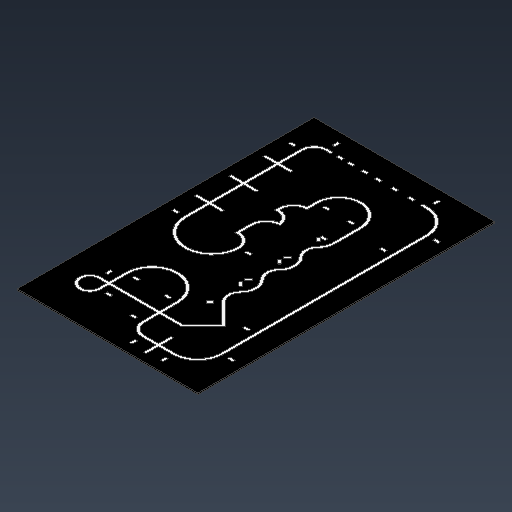
# Autodesk Inventor part: Pista_Teste_V1
Saved by Autodesk Inventor 2026.1 (Build 301233020, 233B)
## iProperties
Created: 2026-04-30
Part Number: Pista_Teste_V1
Material: Genérico
Document SubType Name: Modeling
Designer: celio
Density: 1 g/cm^3
Appearance: Padrão
Author: celio
Autodesk Inventor part; units mm, degrees
ref_plane "YZ Plane" through (0, 0, 0) normal (1, 0, 0) x (0, 1, 0)
ref_plane "XZ Plane" through (0, 0, 0) normal (0, 1, 0) x (-1, 0, 0)
ref_plane "XY Plane" through (0, 0, 0) normal (0, 0, 1) x (1, 0, 0)
sketch "Esboço1" plane through (0, 0, 0) normal (0, 1, 0) x (-1, 0, 0)
  line L0 (0, 0) -> (1320, 0)
  line L1 (1320, 0) -> (1320, -2170)
  line L2 (1320, -2170) -> (0, -2170)
  line L3 (0, -2170) -> (0, 0)
  line L4 (1170, -2020) -> (1170, -150) construction
  line L5 (1170, -150) -> (150, -150) construction
  line L6 (150, -150) -> (150, -2020) construction
  line L7 (150, -2020) -> (1170, -2020) construction
  line L8 (150, -335) -> (150, -1835)
  arc A0 (335, -150) -> (150, -335) centre (335, -335) ccw
  line L9 (150, -335) -> (335, -335) construction
  line L10 (335, -150) -> (335, -335) construction
  arc A1 (660, -250) -> (560, -150) centre (560, -250) ccw
  line L11 (560, -150) -> (560, -250) construction
  line L12 (660, -250) -> (560, -250) construction
  arc A2 (660, -500) -> (1010, -500) centre (835, -500) ccw
  line L13 (660, -500) -> (835, -500) construction
  line L14 (1010, -500) -> (835, -500) construction
  arc A3 (1090, -380) -> (1010, -300) centre (1090, -300) ccw
  line L15 (1010, -300) -> (1090, -300) construction
  line L16 (1090, -380) -> (1090, -300) construction
  line L17 (490, -380) -> (348.5786, -521.4214)
  line L18 (348.5786, -521.4214) -> (490, -662.8427)
  arc A4 (490, -804.2641) -> (490, -662.8427) centre (419.2893, -733.5534) ccw
  line L19 (490, -662.8427) -> (419.2893, -733.5534) construction
  line L20 (490, -804.2641) -> (419.2893, -733.5534) construction
  arc A5 (490, -804.2641) -> (490, -945.6854) centre (560.7107, -874.9747) ccw
  line L21 (490, -804.2641) -> (560.7107, -874.9747) construction
  line L22 (490, -945.6854) -> (560.7107, -874.9747) construction
  arc A6 (490, -1087.1068) -> (490, -945.6854) centre (419.2893, -1016.3961) ccw
  line L23 (490, -945.6854) -> (419.2893, -1016.3961) construction
  line L24 (490, -1087.1068) -> (419.2893, -1016.3961) construction
  arc A7 (490, -1087.1068) -> (490, -1228.5281) centre (560.7107, -1157.8175) ccw
  line L25 (490, -1087.1068) -> (560.7107, -1157.8175) construction
  line L26 (490, -1228.5281) -> (560.7107, -1157.8175) construction
  arc A8 (490, -1369.9495) -> (490, -1228.5281) centre (419.2893, -1299.2388) ccw
  line L27 (490, -1228.5281) -> (419.2893, -1299.2388) construction
  line L28 (490, -1369.9495) -> (419.2893, -1299.2388) construction
  arc A9 (490, -1369.9495) -> (460.7107, -1440.6602) centre (560.7107, -1440.6602) ccw
  line L29 (490, -1369.9495) -> (560.7107, -1440.6602) construction
  line L30 (460.7107, -1440.6602) -> (560.7107, -1440.6602) construction
  line L31 (460.7107, -1440.6602) -> (460.7107, -1640.6602)
  arc A10 (460.7107, -1640.6602) -> (760.7096, -1640.0838) centre (610.7107, -1640.6602) ccw
  arc A11 (1170.7096, -1070.0838) -> (760.7096, -1070.0838) centre (965.7096, -1070.0838) ccw
  line L32 (760.7096, -1070.0838) -> (965.7096, -1070.0838) construction
  line L33 (1170.7096, -1070.0838) -> (965.7096, -1070.0838) construction
  arc A12 (1069.9166, -2020) -> (1170, -1920.0835) centre (1070, -1920) ccw
  line L34 (1170, -1920.0835) -> (1070, -1920) construction
  line L35 (1069.9166, -2020) -> (1070, -1920) construction
  arc A13 (150, -1835) -> (335, -2020) centre (335, -1835) ccw
  line L36 (150, -1835) -> (335, -1835) construction
  line L37 (335, -2020) -> (335, -1835) construction
  line L38 (760.7096, -1640.0838) -> (760.7096, -1560.0838)
  arc A14 (760.7096, -1560.0838) -> (860.7096, -1460.0838) centre (760.7096, -1460.0838) ccw
  arc A15 (760.7096, -1360.0838) -> (860.7096, -1460.0838) centre (860.7096, -1360.0838) ccw
  arc A16 (760.7096, -1360.0838) -> (860.7096, -1260.0838) centre (760.7096, -1260.0838) ccw
  arc A17 (760.7096, -1070.0838) -> (860.7096, -1170.0838) centre (860.7096, -1070.0838) ccw
  line L39 (860.7096, -1170.0838) -> (860.7096, -1260.0838)
  line L40 (1069.9166, -2020) -> (1029.9166, -2020)
  line L41 (1029.9166, -2020) -> (989.9166, -2020) construction
  line L42 (989.9166, -2020) -> (949.9166, -2020)
  line L43 (949.9166, -2020) -> (909.9166, -2020) construction
  line L44 (909.9166, -2020) -> (869.9166, -2020)
  line L45 (869.9166, -2020) -> (809.9166, -2020) construction
  line L46 (809.9166, -2020) -> (769.9166, -2020)
  line L47 (769.9166, -2020) -> (709.9166, -2020) construction
  line L48 (709.9166, -2020) -> (669.9166, -2020)
  line L49 (669.9166, -2020) -> (589.9166, -2020) construction
  line L50 (589.9166, -2020) -> (549.9166, -2020)
  line L51 (549.9166, -2020) -> (469.9166, -2020) construction
  line L52 (469.9166, -2020) -> (429.9166, -2020)
  line L53 (335, -2020) -> (375, -2020)
  line L54 (375, -2000) -> (335, -2000)
  arc A18 (170, -1835) -> (335, -2000) centre (335, -1835) ccw
  line L55 (170, -1835) -> (170, -335)
  arc A19 (335, -170) -> (170, -335) centre (335, -335) ccw
  arc A20 (640, -250) -> (560, -170) centre (560, -250) ccw
  arc A21 (640, -500) -> (1030, -500) centre (835, -500) ccw
  arc A22 (1090, -360) -> (1030, -300) centre (1090, -300) ccw
  line L56 (481.7157, -360) -> (320.2944, -521.4214)
  line L57 (320.2944, -521.4214) -> (475.8579, -676.9848)
  arc A23 (475.8579, -790.1219) -> (475.8579, -676.9848) centre (419.2893, -733.5534) ccw
  arc A24 (475.8579, -790.1219) -> (475.8579, -959.8276) centre (560.7107, -874.9747) ccw
  arc A25 (475.8579, -1072.9646) -> (475.8579, -959.8276) centre (419.2893, -1016.3961) ccw
  arc A26 (475.8579, -1072.9646) -> (475.8579, -1242.6703) centre (560.7107, -1157.8175) ccw
  arc A27 (475.8579, -1355.8074) -> (475.8579, -1242.6703) centre (419.2893, -1299.2388) ccw
  arc A28 (475.8579, -1355.8074) -> (440.7107, -1440.6602) centre (560.7107, -1440.6602) ccw
  line L58 (440.7107, -1440.6602) -> (440.7107, -1640.6602)
  arc A29 (440.7107, -1640.6602) -> (780.7096, -1640.0466) centre (610.7107, -1640.6602) ccw
  line L59 (780.7096, -1640.0466) -> (780.7096, -1578.4054)
  arc A30 (780.7096, -1578.4054) -> (878.6679, -1438.0421) centre (760.7096, -1460.0838) ccw
  arc A31 (782.7513, -1378.0421) -> (878.6679, -1438.0421) centre (860.7096, -1360.0838) ccw
  arc A32 (782.7513, -1378.0421) -> (880.7096, -1260.0838) centre (760.7096, -1260.0838) ccw
  line L60 (880.7096, -1260.0838) -> (880.7096, -1147.5435)
  arc A33 (780.7096, -1070.0838) -> (880.7096, -1147.5435) centre (860.7096, -1070.0838) ccw
  arc A34 (1150.7096, -1070.0757) -> (780.7096, -1070.0838) centre (965.7096, -1070.0838) ccw
  arc A35 (1069.9254, -2000) -> (1150, -1920.0668) centre (1070, -1920) ccw
  line L61 (1069.9254, -2000) -> (1029.9166, -2000)
  line L62 (989.9166, -2000) -> (949.9166, -2000)
  line L63 (909.9166, -2000) -> (869.9166, -2000)
  line L64 (809.9166, -2000) -> (769.9166, -2000)
  line L65 (709.9166, -2000) -> (669.9166, -2000)
  line L66 (589.9166, -2000) -> (549.9166, -2000)
  line L67 (469.9166, -2000) -> (429.9166, -2000)
  line L68 (1029.9166, -2000) -> (1029.9166, -2020)
  line L69 (989.9166, -2000) -> (989.9166, -2020)
  line L70 (949.9166, -2020) -> (949.9166, -2000)
  line L71 (909.9166, -2020) -> (909.9166, -2000)
  line L72 (869.9166, -2020) -> (869.9166, -2000)
  line L73 (809.9166, -2020) -> (809.9166, -2000)
  line L74 (769.9166, -2020) -> (769.9166, -2000)
  line L75 (709.9166, -2020) -> (709.9166, -2000)
  line L76 (669.9166, -2000) -> (669.9166, -2020)
  line L77 (589.9166, -2020) -> (589.9166, -2000)
  line L78 (549.9166, -2000) -> (549.9166, -2020)
  line L79 (469.9166, -2020) -> (469.9166, -2000)
  line L80 (429.9166, -2000) -> (429.9166, -2020)
  line L81 (375, -2020) -> (375, -2000)
  line L82 (1030, -500) -> (1030, -380)
  line L83 (1030, -360) -> (1030, -300)
  line L84 (1010, -500) -> (1010, -380)
  line L85 (1010, -360) -> (1010, -300)
  line L86 (1090, -360) -> (1030, -360)
  line L87 (1090, -380) -> (1030, -380)
  line L88 (660, -250) -> (660, -360)
  line L89 (660, -380) -> (660, -500)
  line L90 (640, -250) -> (640, -360)
  line L91 (640, -380) -> (640, -500)
  line L92 (1010, -360) -> (660, -360)
  line L93 (640, -360) -> (481.7157, -360)
  line L94 (1010, -380) -> (660, -380)
  line L95 (640, -380) -> (490, -380)
  line L96 (490, -380) -> (640, -380) construction
  line L97 (660, -380) -> (690, -380) construction
  line L98 (437.5, -60) -> (457.5, -60)
  line L99 (457.5, -260) -> (437.5, -260)
  line L100 (335, -150) -> (437.5, -150)
  line L101 (457.5, -150) -> (560, -150)
  line L102 (457.5, -60) -> (457.5, -150)
  line L103 (457.5, -170) -> (457.5, -260)
  line L104 (335, -170) -> (437.5, -170)
  line L105 (457.5, -170) -> (560, -170)
  line L106 (437.5, -260) -> (437.5, -170)
  line L107 (437.5, -150) -> (437.5, -60)
  line L108 (1259.948, -1505.075) -> (1259.948, -1485.075)
  line L109 (1059.948, -1485.075) -> (1059.948, -1505.075)
  line L110 (1170.7096, -1070.0838) -> (1170.3631, -1485.075)
  line L111 (1259.948, -1485.075) -> (1170.3631, -1485.075)
  line L112 (1150.3631, -1485.075) -> (1059.948, -1485.075)
  line L113 (1059.948, -1505.075) -> (1150.3464, -1505.075)
  line L114 (1170.3464, -1505.075) -> (1259.948, -1505.075)
  line L115 (1259.7393, -1755.0749) -> (1259.7393, -1735.0749)
  line L116 (1259.7393, -1735.0749) -> (1170.1544, -1735.0749)
  line L117 (1170.1377, -1755.0749) -> (1259.7393, -1755.0749)
  line L118 (1059.7393, -1755.0749) -> (1150.1377, -1755.0749)
  line L119 (1150.1544, -1735.0749) -> (1059.7393, -1735.0749)
  line L120 (1059.7393, -1735.0749) -> (1059.7393, -1755.0749)
  line L121 (1260.1567, -1255.0751) -> (1260.1567, -1235.0751)
  line L122 (1260.1567, -1235.0751) -> (1170.5718, -1235.0751)
  line L123 (1170.5551, -1255.0751) -> (1260.1567, -1255.0751)
  line L124 (1060.1567, -1255.0751) -> (1150.5551, -1255.0751)
  line L125 (1150.5718, -1235.0751) -> (1060.1567, -1235.0751)
  line L126 (1060.1567, -1235.0751) -> (1060.1567, -1255.0751)
  line L127 (1150.7096, -1070.0757) -> (1150.5718, -1235.0751)
  line L128 (1150.5551, -1255.0751) -> (1150.3631, -1485.075)
  line L129 (1150.3464, -1505.075) -> (1150.1544, -1735.0749)
  line L130 (1150.1377, -1755.0749) -> (1150, -1920.0668)
  line L131 (1170.3464, -1505.075) -> (1170.1544, -1735.0749)
  line L132 (1170.1377, -1755.0749) -> (1170, -1920.0835)
  line L133 (110, -325) -> (70, -325)
  line L134 (70, -325) -> (70, -345)
  line L135 (70, -345) -> (110, -345)
  line L136 (110, -345) -> (110, -325)
  line L137 (110, -325) -> (70, -345) construction
  line L138 (70, -325) -> (110, -345) construction
  line L139 (325, -110) -> (345, -110)
  line L140 (345, -110) -> (345, -70)
  line L141 (345, -70) -> (325, -70)
  line L142 (325, -70) -> (325, -110)
  line L143 (325, -110) -> (345, -70) construction
  line L144 (345, -110) -> (325, -70) construction
  line L145 (550, -110) -> (570, -110)
  line L146 (570, -110) -> (570, -70)
  line L147 (570, -70) -> (550, -70)
  line L148 (550, -70) -> (550, -110)
  line L149 (550, -110) -> (570, -70) construction
  line L150 (570, -110) -> (550, -70) construction
  line L151 (700, -260) -> (740, -260)
  line L152 (740, -260) -> (740, -240)
  line L153 (740, -240) -> (700, -240)
  line L154 (700, -240) -> (700, -260)
  line L155 (700, -260) -> (740, -240) construction
  line L156 (740, -260) -> (700, -240) construction
  line L157 (700, -510) -> (740, -510)
  line L158 (740, -510) -> (740, -490)
  line L159 (740, -490) -> (700, -490)
  line L160 (700, -490) -> (700, -510)
  line L161 (700, -510) -> (740, -490) construction
  line L162 (740, -510) -> (700, -490) construction
  line L163 (930, -510) -> (970, -510)
  line L164 (970, -510) -> (970, -490)
  line L165 (970, -490) -> (930, -490)
  line L166 (930, -490) -> (930, -510)
  line L167 (930, -510) -> (970, -490) construction
  line L168 (970, -510) -> (930, -490) construction
  line L169 (930, -310) -> (970, -310)
  line L170 (970, -310) -> (970, -290)
  line L171 (970, -290) -> (930, -290)
  line L172 (930, -290) -> (930, -310)
  line L173 (930, -310) -> (970, -290) construction
  line L174 (970, -310) -> (930, -290) construction
  line L175 (1080, -420) -> (1100, -420)
  line L176 (1100, -420) -> (1100, -460)
  line L177 (1100, -460) -> (1080, -460)
  line L178 (1080, -460) -> (1080, -420)
  line L179 (1080, -420) -> (1100, -460) construction
  line L180 (1100, -420) -> (1080, -460) construction
  line L181 (525.3553, -641.6295) -> (553.6396, -613.3452)
  line L182 (553.6396, -613.3452) -> (539.4975, -599.2031)
  line L183 (539.4975, -599.2031) -> (511.2132, -627.4874)
  line L184 (511.2132, -627.4874) -> (525.3553, -641.6295)
  line L185 (525.3553, -641.6295) -> (539.4975, -599.2031) construction
  line L186 (553.6396, -613.3452) -> (511.2132, -627.4874) construction
  line L187 (525.3553, -825.4773) -> (553.6396, -853.7615)
  line L188 (553.6396, -853.7615) -> (539.4975, -867.9037)
  line L189 (539.4975, -867.9037) -> (511.2132, -839.6194)
  line L190 (511.2132, -839.6194) -> (525.3553, -825.4773)
  line L191 (525.3553, -825.4773) -> (539.4975, -867.9037) construction
  line L192 (553.6396, -853.7615) -> (511.2132, -839.6194) construction
  line L193 (511.2132, -910.3301) -> (539.4975, -882.0458)
  line L194 (539.4975, -882.0458) -> (553.6396, -896.188)
  line L195 (553.6396, -896.188) -> (525.3553, -924.4722)
  line L196 (525.3553, -924.4722) -> (511.2132, -910.3301)
  line L197 (511.2132, -910.3301) -> (553.6396, -896.188) construction
  line L198 (539.4975, -882.0458) -> (525.3553, -924.4722) construction
  line L199 (525.3553, -1108.32) -> (553.6396, -1136.6043)
  line L200 (553.6396, -1136.6043) -> (539.4975, -1150.7464)
  line L201 (539.4975, -1150.7464) -> (511.2132, -1122.4621)
  line L202 (511.2132, -1122.4621) -> (525.3553, -1108.32)
  line L203 (525.3553, -1108.32) -> (539.4975, -1150.7464) construction
  line L204 (553.6396, -1136.6043) -> (511.2132, -1122.4621) construction
  line L205 (511.2132, -1193.1728) -> (539.4975, -1164.8885)
  line L206 (539.4975, -1164.8885) -> (553.6396, -1179.0307)
  line L207 (553.6396, -1179.0307) -> (525.3553, -1207.3149)
  line L208 (525.3553, -1207.3149) -> (511.2132, -1193.1728)
  line L209 (511.2132, -1193.1728) -> (553.6396, -1179.0307) construction
  line L210 (539.4975, -1164.8885) -> (525.3553, -1207.3149) construction
  line L211 (511.2132, -1405.3048) -> (539.4975, -1433.5891)
  line L212 (539.4975, -1433.5891) -> (553.6396, -1419.447)
  line L213 (553.6396, -1419.447) -> (525.3553, -1391.1627)
  line L214 (525.3553, -1391.1627) -> (511.2132, -1405.3048)
  line L215 (511.2132, -1405.3048) -> (553.6396, -1419.447) construction
  line L216 (539.4975, -1433.5891) -> (525.3553, -1391.1627) construction
  line L217 (500.7107, -1430.6602) -> (540.7107, -1430.6602)
  line L218 (540.7107, -1430.6602) -> (540.7107, -1450.6602)
  line L219 (540.7107, -1450.6602) -> (500.7107, -1450.6602)
  line L220 (500.7107, -1450.6602) -> (500.7107, -1430.6602)
  line L221 (500.7107, -1430.6602) -> (540.7107, -1450.6602) construction
  line L222 (540.7107, -1430.6602) -> (500.7107, -1450.6602) construction
  line L223 (540.7107, -1630.0466) -> (500.7107, -1630.0466)
  line L224 (500.7107, -1630.0466) -> (500.7107, -1650.0466)
  line L225 (500.7107, -1650.0466) -> (540.7107, -1650.0466)
  line L226 (540.7107, -1650.0466) -> (540.7107, -1630.0466)
  line L227 (540.7107, -1630.0466) -> (500.7107, -1650.0466) construction
  line L228 (500.7107, -1630.0466) -> (540.7107, -1650.0466) construction
  line L229 (680.7096, -1630.0466) -> (720.7096, -1630.0466)
  line L230 (720.7096, -1630.0466) -> (720.7096, -1650.0466)
  line L231 (720.7096, -1650.0466) -> (680.7096, -1650.0466)
  line L232 (680.7096, -1650.0466) -> (680.7096, -1630.0466)
  line L233 (680.7096, -1630.0466) -> (720.7096, -1650.0466) construction
  line L234 (720.7096, -1630.0466) -> (680.7096, -1650.0466) construction
  line L235 (720.7096, -1060.0838) -> (680.7096, -1060.0838)
  line L236 (680.7096, -1060.0838) -> (680.7096, -1080.0838)
  line L237 (680.7096, -1080.0838) -> (720.7096, -1080.0838)
  line L238 (720.7096, -1080.0838) -> (720.7096, -1060.0838)
  line L239 (720.7096, -1060.0838) -> (680.7096, -1080.0838) construction
  line L240 (680.7096, -1060.0838) -> (720.7096, -1080.0838) construction
  line L241 (1210.7096, -1080.0838) -> (1250.7096, -1080.0838)
  line L242 (1250.7096, -1080.0838) -> (1250.7096, -1060.0838)
  line L243 (1250.7096, -1060.0838) -> (1210.7096, -1060.0838)
  line L244 (1210.7096, -1060.0838) -> (1210.7096, -1080.0838)
  line L245 (1210.7096, -1080.0838) -> (1250.7096, -1060.0838) construction
  line L246 (1250.7096, -1080.0838) -> (1210.7096, -1060.0838) construction
  line L247 (1250, -1930.1167) -> (1210, -1930.1167)
  line L248 (1210, -1930.1167) -> (1210, -1910.1167)
  line L249 (1210, -1910.1167) -> (1250, -1910.1167)
  line L250 (1250, -1910.1167) -> (1250, -1930.1167)
  line L251 (1250, -1930.1167) -> (1210, -1910.1167) construction
  line L252 (1210, -1930.1167) -> (1250, -1910.1167) construction
  line L253 (1059.8811, -2060) -> (1079.8811, -2060)
  line L254 (1079.8811, -2060) -> (1079.8811, -2100)
  line L255 (1079.8811, -2100) -> (1059.8811, -2100)
  line L256 (1059.8811, -2100) -> (1059.8811, -2060)
  line L257 (1059.8811, -2060) -> (1079.8811, -2100) construction
  line L258 (1079.8811, -2060) -> (1059.8811, -2100) construction
  line L259 (325, -2060) -> (345, -2060)
  line L260 (345, -2060) -> (345, -2100)
  line L261 (345, -2100) -> (325, -2100)
  line L262 (325, -2100) -> (325, -2060)
  line L263 (325, -2060) -> (345, -2100) construction
  line L264 (345, -2060) -> (325, -2100) construction
  line L265 (110, -1825) -> (70, -1825)
  line L266 (70, -1825) -> (70, -1845)
  line L267 (70, -1845) -> (110, -1845)
  line L268 (110, -1845) -> (110, -1825)
  line L269 (110, -1825) -> (70, -1845) construction
  line L270 (70, -1825) -> (110, -1845) construction
  line L271 (170, -1085) -> (270, -1085) construction
  line L272 (250, -575) -> (210, -575)
  line L273 (210, -575) -> (210, -595)
  line L274 (210, -595) -> (250, -595)
  line L275 (250, -595) -> (250, -575)
  line L276 (250, -575) -> (210, -595) construction
  line L277 (210, -575) -> (250, -595) construction
  line L278 (250, -1575) -> (210, -1575)
  line L279 (210, -1575) -> (210, -1595)
  line L280 (210, -1595) -> (250, -1595)
  line L281 (250, -1595) -> (250, -1575)
  line L282 (250, -1575) -> (210, -1595) construction
  line L283 (210, -1575) -> (250, -1595) construction
  point P0 (150, -1085)
  point P1 (447.5, -150)
  point P2 (1170.3548, -1495.0837)
  point P3 (447.5, -160)
  point P4 (1159.948, -1495.075)
  point P5 (90, -335)
  point P6 (335, -90)
  point P7 (560, -90)
  point P8 (720, -250)
  point P9 (720, -500)
  point P10 (950, -500)
  point P11 (950, -300)
  point P12 (1090, -440)
  point P13 (532.4264, -620.4163)
  point P14 (532.4264, -846.6905)
  point P15 (532.4264, -903.259)
  point P16 (532.4264, -1129.5332)
  point P17 (532.4264, -1186.1017)
  point P18 (532.4264, -1412.3759)
  point P19 (520.7107, -1440.6602)
  point P20 (520.7107, -1640.0466)
  point P21 (700.7096, -1640.0466)
  point P22 (700.7096, -1070.0838)
  point P23 (1230.7096, -1070.0838)
  point P24 (1230, -1920.1167)
  point P25 (1069.8811, -2080)
  point P26 (335, -2080)
  point P27 (90, -1835)
  point P28 (230, -585)
  point P29 (230, -1585)
  point P30 (536.5685, -1430.6602)
  point P31 (540.7107, -1432.3759)
  dimension "d0" = 1320
  dimension "d1" = 2170
  dimension "d2" = 150
  dimension "d3" = 1500
  dimension "d4" = 185
  dimension "d5" = 90
  dimension "d7" = 225
  dimension "d8" = 100
  dimension "d9" = 90
  dimension "d10" = 250
  dimension "d11" = 175
  dimension "d12" = 180
  dimension "d13" = 200
  dimension "d14" = 80
  dimension "d15" = 270
  dimension "d16" = 600
  dimension "d17" = 200
  dimension "d19" = 200
  dimension "d20" = 90
  dimension "d21" = 100
  dimension "d22" = 90
  dimension "d23" = 100
  dimension "d24" = 90
  dimension "d25" = 100
  dimension "d26" = 90
  dimension "d27" = 100
  dimension "d28" = 90
  dimension "d29" = 100
  dimension "d30" = 90
  dimension "d31" = 100
  dimension "d32" = 45
  dimension "d33" = 200
  dimension "d34" = 150
  dimension "d35" = 570
  dimension "d36" = 205
  dimension "d37" = 180
  dimension "d38" = 850
  dimension "d39" = 100
  dimension "d40" = 90
  dimension "d41" = 185
  dimension "d42" = 90
  dimension "d43" = 80
  dimension "d46" = 100
  dimension "d49" = 100
  dimension "d52" = 100
  dimension "d55" = 100
  dimension "d56" = 90
  dimension "d57" = 40
  dimension "d58" = 40
  dimension "d59" = 40
  dimension "d60" = 40
  dimension "d61" = 40
  dimension "d62" = 60
  dimension "d63" = 40
  dimension "d64" = 60
  dimension "d65" = 40
  dimension "d66" = 80
  dimension "d67" = 40
  dimension "d68" = 80
  dimension "d69" = 40
  dimension "d70" = 40
  dimension "d71" = 54.9166
  dimension "d82" = 20
  dimension "d83" = 20
  constraints: 566 end point, 79 parallel, 72 point on circle, 53 midpoint, 38 perpendicular, 36 centre point, 30 horizontal, 18 tangent, 17 point on line, 6 vertical, 69 other
  measures "d0" distance of L1.end L2.end
  measures "d1" distance of L0.end L1.end
  measures "d2" distance between parallel lines of L1 L4
  measures "d3" distance of L8.start L8.end
  measures "d4" radius of A0
  measures "d5" angle of L10 L9
  measures "d7" distance of L10.start L11.start
  measures "d8" radius of A1
  measures "d9" angle of L12 L11
  measures "d10" distance of L12.start L13.start
  measures "d11" radius of A2
  measures "d12" angle of L13 L14
  measures "d13" distance of L14.start L15.start
  measures "d14" radius of A3
  measures "d16" distance of L16.start L17.start
  measures "d17" distance of L17.start L17.end
  measures "d19" distance of L17.end L18.end
  measures "d20" angle of L18 L17
  measures "d21" radius of A4
  measures "d22" angle of L20 L19
  measures "d23" radius of A5
  measures "d24" angle of L21 L22
  measures "d25" radius of A6
  measures "d26" angle of L24 L23
  measures "d27" radius of A7
  measures "d28" angle of L25 L26
  measures "d29" radius of A8
  measures "d30" angle of L28 L27
  measures "d31" radius of A9
  measures "d32" angle of L29 L30
  measures "d33" distance of L30.start L31.end
  measures "d34" radius of A10
  measures "d35" distance of L38.start L32.start
  measures "d36" radius of A11
  measures "d37" angle of L32 L33
  measures "d38" distance of L33.start L34.start
  measures "d39" radius of A12
  measures "d40" angle of L35 L34
  measures "d41" radius of A13
  measures "d42" angle of L36 L37
  measures "d43" distance of L38.start L38.end
  measures "d46" radius of A14
  measures "d49" radius of A15
  measures "d52" radius of A16
  measures "d55" radius of A17
  measures "d56" distance of L39.start L39.end
  measures "d57" distance of L35.start L40.end
  measures "d58" distance of L40.end L41.end
  measures "d59" distance of L41.end L42.end
  measures "d60" distance of L42.end L43.end
  measures "d61" distance of L43.end L44.end
  measures "d62" distance of L44.end L45.end
  measures "d63" distance of L45.end L46.end
  measures "d64" distance of L46.end L47.end
  measures "d65" distance of L47.end L48.end
  measures "d66" distance of L48.end L49.end
  measures "d67" distance of L49.end L50.end
  measures "d68" distance of L50.end L51.end
  measures "d69" distance of L51.end L52.end
  measures "d70" distance of L37.start L53.end
  measures "d71" distance of L53.end L52.end
  measures "d82" distance between parallel lines of L8 L55
  measures "d83" distance of L99.start L99.end
extrude "Extrusão1" add sketch "Esboço1" along normal blind 0.1 contours A0 L100 L107 L98 L102 L101 A1 L88 L92 L85 A3 L87 L82 A21 L91 L95 L17 L18 A4 A5 A6 A7 A8 A9 L31 A10 L38 A14 A15 A16 L39 A17 A11 L110 L111 L108 L114 L131 L116 L115 L117 L132 A12 L40 L68 L61 A35 L130 L118 L120 L119 L129 L113 L109 L112 L128 L124 L126 L125 L127 A34 A33 L60 A32 A31 A30 L59 A29 L58 A28 A27 A26 A25 A24 A23 L57 L56 L93 L90 A20 L105 L103 L99 L106 L104 A19 L55 A18 L54 L81 L53 A13 L8 | L122 L121 L123 L110 | L42 L70 L62 L69 | L44 L72 L63 L71 | L46 L74 L64 L73 | L48 L76 L65 L75 | L50 L78 L66 L77 | L52 L80 L67 L79
extrude "Extrusão2" add sketch "Esboço1" against normal blind 10 contours L0 L1 L2 L3 | A0 L100 L107 L98 L102 L101 A1 L88 L92 L85 A3 L87 L82 A21 L91 L95 L17 L18 A4 A5 A6 A7 A8 A9 L31 A10 L38 A14 A15 A16 L39 A17 A11 L110 L111 L108 L114 L131 L116 L115 L117 L132 A12 L40 L68 L61 A35 L130 L118 L120 L119 L129 L113 L109 L112 L128 L124 L126 L125 L127 A34 A33 L60 A32 A31 A30 L59 A29 L58 A28 A27 A26 A25 A24 A23 L57 L56 L93 L90 A20 L105 L103 L99 L106 L104 A19 L55 A18 L54 L81 L53 A13 L8 | L122 L121 L123 L110 | L89 L94 L84 A2 | L42 L70 L62 L69 | L44 L72 L63 L71 | L46 L74 L64 L73 | L48 L76 L65 L75 | L50 L78 L66 L77 | L52 L80 L67 L79 | L86 L83 A22 | L136 L135 L134 L133 | L142 L141 L140 L139 | L148 L147 L146 L145 | L154 L153 L152 L151 | L160 L159 L158 L157 | L166 L165 L164 L163 | L172 L171 L170 L169 | L175 L176 L177 L178 | L184 L183 L182 L181 | L187 L188 L189 L190 | L193 L194 L195 L196 | L199 L200 L201 L202 | L205 L206 L207 L208 | L214 L213 L212 L218 L217 L211 | L217 L218 L212 L211 | L211 L212 L218 L219 L220 L217 | L226 L225 L224 L223 | L229 L230 L231 L232 | L238 L237 L236 L235 | L244 L243 L242 L241 | L247 L248 L249 L250 | L253 L254 L255 L256 | L259 L260 L261 L262 | L268 L267 L266 L265 | L275 L274 L273 L272 | L281 L280 L279 L278
extrude "Extrusão3" add sketch "Esboço1" along normal blind 0.1 contours L136 L135 L134 L133 | L142 L141 L140 L139 | L148 L147 L146 L145 | L154 L153 L152 L151 | L160 L159 L158 L157 | L166 L165 L164 L163 | L172 L171 L170 L169 | L175 L176 L177 L178 | L184 L183 L182 L181 | L187 L188 L189 L190 | L193 L194 L195 L196 | L199 L200 L201 L202 | L205 L206 L207 L208 | L214 L213 L212 L218 L217 L211 | L217 L218 L212 L211 | L211 L212 L218 L219 L220 L217 | L226 L225 L224 L223 | L229 L230 L231 L232 | L238 L237 L236 L235 | L244 L243 L242 L241 | L247 L248 L249 L250 | L253 L254 L255 L256 | L259 L260 L261 L262 | L268 L267 L266 L265 | L275 L274 L273 L272 | L281 L280 L279 L278
